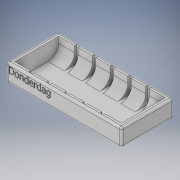
# Autodesk Inventor part: bakje woensdag
Saved by Autodesk Inventor 2019 (Build 230136000, 136)
## iProperties
Created: 2020-10-20
Part Number: bakje woensdag
Material: Generic
Document SubType Name: Modeling
Designer: daanswinters
Density: 1 g/cm^3
Appearance: Default
Author: daanswinters
Autodesk Inventor part; units mm, degrees
ref_plane "YZ Plane" through (0, 0, 0) normal (1, 0, 0) x (0, 1, 0)
ref_plane "XZ Plane" through (0, 0, 0) normal (0, 1, 0) x (-1, 0, 0)
ref_plane "XY Plane" through (0, 0, 0) normal (0, 0, 1) x (1, 0, 0)
sketch "Sketch1" plane through (0, 0, 0) normal (0, 0, 1) x (1, 0, 0)
  line L0 (55, -8.5) -> (-55, -8.5)
  line L1 (-55, -8.5) -> (-55, 8.5)
  line L2 (-55, 8.5) -> (55, 8.5)
  line L3 (55, 8.5) -> (55, -8.5)
  line L4 (55, -8.5) -> (-55, 8.5) construction
  line L5 (-55, -8.5) -> (55, 8.5) construction
  point P0 (0, 0)
  dimension "d0" = 110
  dimension "d1" = 17
  constraints: 12 end point, 2 midpoint, 2 parallel, 1 horizontal, 1 perpendicular
  measures "d0" distance of L1.end L2.end
  measures "d1" distance of L0.end L1.end
extrude "Extrusion1" add sketch "Sketch1" along normal blind 50
sketch "Sketch2" plane through (-55, 8.5, 0) normal (0, 1, 0) x (1, 0, 0)
  line L0 (0, 0) -> (0, -50) projected
  line L1 (110, -50) -> (0, -50)
  line L2 (0, -50) -> (0, 0)
  line L3 (0, 0) -> (110, 0)
  line L4 (110, 0) -> (110, -50)
  line L5 (110, -50) -> (0, 0) construction
  line L6 (0, -50) -> (110, 0) construction
  line L7 (106, -46) -> (106, -4)
  line L8 (4, -4) -> (4, -46)
  line L9 (56.15, -2) -> (53.85, -2)
  line L10 (53.85, -48) -> (56.15, -48)
  line L11 (56.15, -2) -> (53.85, -48) construction
  line L12 (53.85, -2) -> (56.15, -48) construction
  line L13 (73.15, -2) -> (70.85, -2)
  line L14 (70.85, -48) -> (73.15, -48)
  line L15 (73.15, -2) -> (70.85, -48) construction
  line L16 (70.85, -2) -> (73.15, -48) construction
  line L17 (0, -25) -> (110, -25) construction
  line L18 (87.85, -2) -> (90.15, -2)
  line L19 (90.15, -48) -> (87.85, -48)
  line L20 (87.85, -2) -> (90.15, -48) construction
  line L21 (90.15, -2) -> (87.85, -48) construction
  line L22 (36.85, -2) -> (39.15, -2)
  line L23 (39.15, -48) -> (36.85, -48)
  line L24 (36.85, -2) -> (39.15, -48) construction
  line L25 (39.15, -2) -> (36.85, -48) construction
  line L26 (19.85, -2) -> (22.15, -2)
  line L27 (22.15, -48) -> (19.85, -48)
  line L28 (19.85, -2) -> (22.15, -48) construction
  line L29 (22.15, -2) -> (19.85, -48) construction
  line L30 (90.15, -2) -> (90.15, -4)
  line L31 (90.15, -46) -> (90.15, -48)
  line L32 (87.85, -48) -> (87.85, -46)
  line L33 (87.85, -4) -> (87.85, -2)
  line L34 (73.15, -48) -> (73.15, -46)
  line L35 (73.15, -4) -> (73.15, -2)
  line L36 (70.85, -2) -> (70.85, -4)
  line L37 (70.85, -46) -> (70.85, -48)
  line L38 (56.15, -4) -> (56.15, -2)
  line L39 (53.85, -2) -> (53.85, -4)
  line L40 (53.85, -46) -> (53.85, -48)
  line L41 (56.15, -48) -> (56.15, -46)
  line L42 (39.15, -2) -> (39.15, -4)
  line L43 (39.15, -46) -> (39.15, -48)
  line L44 (36.85, -48) -> (36.85, -46)
  line L45 (36.85, -4) -> (36.85, -2)
  line L46 (22.15, -2) -> (22.15, -4)
  line L47 (19.85, -48) -> (19.85, -46)
  line L48 (19.85, -4) -> (19.85, -2)
  line L49 (22.15, -46) -> (22.15, -48)
  line L50 (4, -46) -> (19.95, -46)
  line L51 (22.05, -46) -> (36.95, -46)
  line L52 (39.05, -46) -> (53.95, -46)
  line L53 (56.05, -46) -> (70.95, -46)
  line L54 (73.05, -46) -> (87.95, -46)
  line L55 (90.05, -46) -> (106, -46)
  line L56 (106, -4) -> (90.05, -4)
  line L57 (87.95, -4) -> (73.05, -4)
  line L58 (70.95, -4) -> (56.05, -4)
  line L59 (53.95, -4) -> (39.05, -4)
  line L60 (36.95, -4) -> (22.05, -4)
  line L61 (19.95, -4) -> (4, -4)
  point P0 (55, 0)
  point P1 (55, -25)
  point P2 (72, -25)
  point P3 (89, -25)
  point P4 (38, -25)
  point P5 (21, -25)
  dimension "d4" = 65.556
  dimension "d5" = 110
  dimension "d7" = 2.3
  dimension "d8" = 46
  dimension "d9" = 2.3
  dimension "d10" = 46
  dimension "d11" = 0
  dimension "d12" = 2.3
  dimension "d13" = 46
  dimension "d14" = 2.3
  dimension "d15" = 46
  dimension "d16" = 2.3
  dimension "d17" = 46
  dimension "d18" = 17
  dimension "d19" = 17
  dimension "d20" = 17
  dimension "d21" = 17
  dimension "d22" = 2.862
  dimension "d23" = 2.862
  dimension "d24" = 106
  dimension "d25" = 4
  dimension "d26" = 42
  dimension "d27" = 2
  dimension "d28" = 0
  dimension "d29" = 42
  dimension "d30" = 0
  dimension "d31" = 42
  dimension "d32" = 0
  dimension "d33" = 42
  dimension "d34" = 0
  dimension "d35" = 42
  dimension "d36" = 0
  dimension "d37" = 42
  constraints: 122 end point, 73 parallel, 43 point on line, 17 perpendicular, 14 midpoint, 6 horizontal
  measures "d4" angle of L5 L0
  measures "d5" distance between parallel lines of L4 L0
  measures "d7" distance of L10.end L10.start
  measures "d8" distance of L10.start L9.end
  measures "d9" distance of L14.end L14.start
  measures "d10" distance of L14.start L13.end
  measures "d11" distance from line of L17 point (72, -25)
  measures "d12" distance of L19.start L19.end
  measures "d13" distance of L18.end L19.start
  measures "d14" distance of L23.start L23.end
  measures "d15" distance of L22.end L23.start
  measures "d16" distance of L27.start L27.end
  measures "d17" distance of L26.end L27.start
  measures "d18" distance of point (72, -25) point (55, -25)
  measures "d19" distance of point (89, -25) point (72, -25)
  measures "d20" distance of point (38, -25) point (55, -25)
  measures "d21" distance of point (21, -25) point (38, -25)
  measures "d22" angle of L0 L20
  measures "d23" angle of L0 L21
  measures "d24" distance between parallel lines of L7 L0
  measures "d25" distance between parallel lines of L8 L0
  measures "d26" distance between parallel lines of L56 L55
  measures "d27" distance between parallel lines of L56 L18
  measures "d28" distance between parallel lines of L56 L57
  measures "d29" distance between parallel lines of L56 L54
  measures "d30" distance between parallel lines of L56 L58
  measures "d31" distance between parallel lines of L56 L53
  measures "d32" distance between parallel lines of L56 L59
  measures "d33" distance between parallel lines of L56 L52
  measures "d34" distance between parallel lines of L56 L60
  measures "d35" distance between parallel lines of L56 L51
  measures "d36" distance between parallel lines of L56 L61
  measures "d37" distance between parallel lines of L56 L50
extrude "Extrusion2" cut sketch "Sketch2" against normal blind 16 contours L55 L31 L19 L32 L54 L34 L14 L37 L53 L41 L10 L40 L52 L43 L23 L44 L51 L49 L27 L47 L50 L8 L61 L48 L26 L46 L60 L45 L22 L42 L59 L39 L9 L38 L58 L36 L13 L35 L57 L33 L18 L30 L56 L7
fillet "Fillet1" radius 2 12 edges at (-55, 0, 50) (-55, 0, 0) (55, 0, 50) (55, 0, 0) (0, 8.5, 50) (-55, 8.5, 25) (0, 8.5, 0) (55, 8.5, 25) (55, -8.5, 25) (0, -8.5, 50) (-55, -8.5, 25) (0, -8.5, 0)
fillet "Fillet2" radius 10 6 edges at (-43.075, -7.5, 4) (-25.5, -7.5, 4) (-8.5, -7.5, 4) (8.5, -7.5, 4) (25.5, -7.5, 4) (43.075, -7.5, 4)
sketch "Sketch3" plane through (35.15, 8.5, 4) normal (0, 1, 0) x (1, 0, 0)
  line L0 (-70.3, -44) -> (-70.3, -42) projected
  line L1 (-51, 2) -> (-53.3, 2)
  line L2 (-34, 2) -> (-34, 0) projected
  line L3 (-36.3, -44) -> (-36.3, -42) projected
  line L4 (-19.3, -44) -> (-19.3, -42) projected
  line L5 (-2.3, -44) -> (-2.3, -42) projected
  line L6 (0, 2) -> (0, 0) projected
  line L7 (-19.8, 2) -> (-16.5, 2)
  line L8 (-16.5, 2) -> (-16.5, -44)
  line L9 (-16.5, -44) -> (-19.8, -44)
  line L10 (-19.8, -44) -> (-19.8, 2)
  line L11 (-19.8, 2) -> (-16.5, -44) construction
  line L12 (-16.5, 2) -> (-19.8, -44) construction
  line L13 (-2.8, -44) -> (0.5, -44)
  line L14 (0.5, -44) -> (0.5, 2)
  line L15 (0.5, 2) -> (-2.8, 2)
  line L16 (-2.8, 2) -> (-2.8, -44)
  line L17 (-2.8, -44) -> (0.5, 2) construction
  line L18 (0.5, -44) -> (-2.8, 2) construction
  line L19 (-36.8, -44) -> (-33.5, -44)
  line L20 (-33.5, -44) -> (-33.5, 2)
  line L21 (-33.5, 2) -> (-36.8, 2)
  line L22 (-36.8, 2) -> (-36.8, -44)
  line L23 (-36.8, -44) -> (-33.5, 2) construction
  line L24 (-33.5, -44) -> (-36.8, 2) construction
  line L25 (-51, 2) -> (-36.3, 2) projected
  line L26 (-53.8, -44) -> (-50.5, -44)
  line L27 (-50.5, -44) -> (-50.5, 2)
  line L28 (-50.5, 2) -> (-53.8, 2)
  line L29 (-53.8, 2) -> (-53.8, -44)
  line L30 (-53.8, -44) -> (-50.5, 2) construction
  line L31 (-50.5, -44) -> (-53.8, 2) construction
  line L32 (-53.3, -44) -> (-68, -44) projected
  line L33 (-70.8, 2) -> (-67.5, 2)
  line L34 (-67.5, 2) -> (-67.5, -44)
  line L35 (-67.5, -44) -> (-70.8, -44)
  line L36 (-70.8, -44) -> (-70.8, 2)
  line L37 (-70.8, 2) -> (-67.5, -44) construction
  line L38 (-67.5, 2) -> (-70.8, -44) construction
  point P0 (-35.15, 4)
  point P1 (-68, 2)
  point P2 (-17, 2)
  point P3 (-18.15, -21)
  point P4 (-1.15, -21)
  point P5 (-35.15, -21)
  point P6 (-52.15, -21)
  point P7 (-69.15, -21)
  dimension "d42" = 3.3
  dimension "d43" = 46
  dimension "d44" = 3.3
  dimension "d45" = 3.3
  dimension "d46" = 3.3
  dimension "d47" = 3.3
  dimension "d48" = 90
  dimension "d49" = 0.5
  dimension "d50" = 16.5
  dimension "d51" = 33.5
  dimension "d52" = 50.5
  dimension "d53" = 67.5
  dimension "d54" = 46
  dimension "d55" = 0
  dimension "d56" = 53.3
  constraints: 62 end point, 14 parallel, 10 midpoint, 5 horizontal, 5 perpendicular, 3 point on line
  measures "d42" distance of L8.end L9.end
  measures "d43" distance of L7.end L8.end
  measures "d44" distance of L15.end L14.end
  measures "d45" distance of L21.end L20.end
  measures "d46" distance of L28.end L27.end
  measures "d47" distance of L34.end L35.end
  measures "d48" angle of L6 L1
  measures "d49" distance between parallel lines of L6 L14
  measures "d50" distance between parallel lines of L6 L8
  measures "d51" distance between parallel lines of L6 L20
  measures "d52" distance between parallel lines of L6 L27
  measures "d53" distance between parallel lines of L6 L34
  measures "d54" distance between parallel lines of L25 L9
  measures "d55" distance between parallel lines of L15 L25
  measures "d56" distance from line of L1.end L6
extrude "Extrusion3" cut sketch "Sketch3" against normal blind 16
sketch "Sketch4" plane through (0, 0, 50) normal (0, 0, 1) x (1, 0, 0)
  line L0 (-52.9749, 6.5012) -> (53.0345, 6.5012) construction
  line L1 (53.0345, 6.5012) -> (53.0345, -6.5247) construction
  line L2 (53.0345, -6.5247) -> (-52.9749, -6.5247) construction
  line L3 (-52.9749, -6.5247) -> (-52.9749, 6.5012) construction
  spline S0 degree 2 poles (-47.5472, 3.1744) (-47.5472, 2.339) (-48.2244, 0.9944) (-48.7929, 0.6188) knots 0 0 0 1 2 2 2
  spline S1 degree 2 poles (-48.7929, 0.6188) (-49.2576, 0.3271) (-50.2116, 0.1294) (-50.9531, 0.1294) knots 0 0 0 1 2 2 2
  line L4 (-50.9531, 0.1294) -> (-52.357, 0.1294)
  line L5 (-52.357, 0.1294) -> (-52.357, 6.2294)
  line L6 (-52.357, 6.2294) -> (-50.968, 6.2294)
  spline S2 degree 2 poles (-50.968, 6.2294) (-50.1078, 6.2294) (-49.1291, 5.9723) (-48.783, 5.7449) knots 0 0 0 1 2 2 2
  spline S3 degree 2 poles (-48.783, 5.7449) (-48.1948, 5.3544) (-47.5472, 4.0642) (-47.5472, 3.1744) knots 0 0 0 1 2 2 2
  spline S4 degree 2 poles (-48.3925, 3.1843) (-48.3925, 3.8863) (-48.8572, 4.8799) (-49.3169, 5.1616) knots 0 0 0 1 2 2 2
  spline S5 degree 2 poles (-49.3169, 5.1616) (-49.6432, 5.3544) (-50.3797, 5.5274) (-50.9284, 5.5274) knots 0 0 0 1 2 2 2
  line L7 (-50.9284, 5.5274) -> (-51.5463, 5.5274)
  line L8 (-51.5463, 5.5274) -> (-51.5463, 0.8313)
  line L9 (-51.5463, 0.8313) -> (-50.9284, 0.8313)
  spline S6 degree 2 poles (-50.9284, 0.8313) (-50.3896, 0.8313) (-49.574, 1.0043) (-49.2428, 1.2367) knots 0 0 0 1 2 2 2
  spline S7 degree 2 poles (-49.2428, 1.2367) (-48.8176, 1.5234) (-48.3925, 2.4725) (-48.3925, 3.1843) knots 0 0 0 1 2 2 2
  spline S8 degree 2 poles (-42.9648, 2.4181) (-42.9648, 1.2614) (-44.077, 0.0008) (-45.0064, 0.0008) knots 0 0 0 1 2 2 2
  spline S9 degree 2 poles (-45.0064, 0.0008) (-45.9604, 0.0008) (-47.0529, 1.3009) (-47.0529, 2.4181) knots 0 0 0 1 2 2 2
  spline S10 degree 2 poles (-47.0529, 2.4181) (-47.0529, 3.5649) (-45.9258, 4.8354) (-45.0064, 4.8354) knots 0 0 0 1 2 2 2
  spline S11 degree 2 poles (-45.0064, 4.8354) (-44.077, 4.8354) (-42.9648, 3.5699) (-42.9648, 2.4181) knots 0 0 0 1 2 2 2
  spline S12 degree 2 poles (-43.7607, 2.4181) (-43.7607, 3.3079) (-44.4082, 4.173) (-45.0064, 4.173) knots 0 0 0 1 2 2 2
  spline S13 degree 2 poles (-45.0064, 4.173) (-45.6045, 4.173) (-46.257, 3.3079) (-46.257, 2.4181) knots 0 0 0 1 2 2 2
  spline S14 degree 2 poles (-46.257, 2.4181) (-46.257, 1.553) (-45.6045, 0.6632) (-45.0064, 0.6632) knots 0 0 0 1 2 2 2
  spline S15 degree 2 poles (-45.0064, 0.6632) (-44.4132, 0.6632) (-43.7607, 1.5382) (-43.7607, 2.4181) knots 0 0 0 1 2 2 2
  line L10 (-38.5801, 0.1294) -> (-39.3513, 0.1294)
  line L11 (-39.3513, 0.1294) -> (-39.3513, 2.7394)
  spline S16 degree 2 poles (-39.3513, 2.7394) (-39.3513, 3.0558) (-39.4106, 3.5995) (-39.4996, 3.7627) knots 0 0 0 1 2 2 2
  spline S17 degree 2 poles (-39.4996, 3.7627) (-39.5935, 3.9357) (-39.9296, 4.1038) (-40.2163, 4.1038) knots 0 0 0 1 2 2 2
  spline S18 degree 2 poles (-40.2163, 4.1038) (-40.503, 4.1038) (-41.1111, 3.7973) (-41.4027, 3.5501) knots 0 0 0 1 2 2 2
  line L12 (-41.4027, 3.5501) -> (-41.4027, 0.1294)
  line L13 (-41.4027, 0.1294) -> (-42.1739, 0.1294)
  line L14 (-42.1739, 0.1294) -> (-42.1739, 4.7068)
  line L15 (-42.1739, 4.7068) -> (-41.4027, 4.7068)
  line L16 (-41.4027, 4.7068) -> (-41.4027, 4.1977)
  spline S19 degree 2 poles (-41.4027, 4.1977) (-41.0567, 4.5091) (-40.3894, 4.8354) (-40.0137, 4.8354) knots 0 0 0 1 2 2 2
  spline S20 degree 2 poles (-40.0137, 4.8354) (-39.3414, 4.8354) (-38.5801, 3.9456) (-38.5801, 3.1003) knots 0 0 0 1 2 2 2
  line L17 (-38.5801, 3.1003) -> (-38.5801, 0.1294)
  line L18 (-33.9779, 0.1294) -> (-34.7491, 0.1294)
  line L19 (-34.7491, 0.1294) -> (-34.7491, 0.594)
  spline S21 degree 2 poles (-34.7491, 0.594) (-34.927, 0.4457) (-35.189, 0.248) (-35.367, 0.164) knots 0 0 0 1 2 2 2
  spline S22 degree 2 poles (-35.367, 0.164) (-35.5301, 0.0849) (-35.8811, 0.0008) (-36.1134, 0.0008) knots 0 0 0 1 2 2 2
  spline S23 degree 2 poles (-36.1134, 0.0008) (-36.4891, 0.0008) (-37.1218, 0.3123) (-37.3443, 0.6138) knots 0 0 0 1 2 2 2
  spline S24 degree 2 poles (-37.3443, 0.6138) (-37.5667, 0.9153) (-37.8139, 1.8051) (-37.8139, 2.3835) knots 0 0 0 1 2 2 2
  spline S25 degree 2 poles (-37.8139, 2.3835) (-37.8139, 2.9866) (-37.5025, 3.8665) (-37.2306, 4.1977) knots 0 0 0 1 2 2 2
  spline S26 degree 2 poles (-37.2306, 4.1977) (-36.9785, 4.4943) (-36.2716, 4.8354) (-35.8811, 4.8354) knots 0 0 0 1 2 2 2
  spline S27 degree 2 poles (-35.8811, 4.8354) (-35.54, 4.8354) (-35.0308, 4.6821) (-34.7491, 4.5239) knots 0 0 0 1 2 2 2
  line L20 (-34.7491, 4.5239) -> (-34.7491, 6.5012)
  line L21 (-34.7491, 6.5012) -> (-33.9779, 6.5012)
  line L22 (-33.9779, 6.5012) -> (-33.9779, 0.1294)
  line L23 (-34.7491, 1.2416) -> (-34.7491, 3.8863)
  spline S28 degree 2 poles (-34.7491, 3.8863) (-35.0358, 4.0247) (-35.4906, 4.1285) (-35.7526, 4.1285) knots 0 0 0 1 2 2 2
  spline S29 degree 2 poles (-35.7526, 4.1285) (-36.3458, 4.1285) (-37.018, 3.2387) (-37.018, 2.3983) knots 0 0 0 1 2 2 2
  spline S30 degree 2 poles (-37.018, 2.3983) (-37.018, 1.5876) (-36.5039, 0.7324) (-35.9355, 0.7324) knots 0 0 0 1 2 2 2
  spline S31 degree 2 poles (-35.9355, 0.7324) (-35.6339, 0.7324) (-35.021, 1.0093) (-34.7491, 1.2416) knots 0 0 0 1 2 2 2
  spline S32 degree 2 poles (-30.8735, 0.0256) (-31.971, 0.0256) (-33.1771, 1.2564) (-33.1771, 2.3934) knots 0 0 0 1 2 2 2
  spline S33 degree 2 poles (-33.1771, 2.3934) (-33.1771, 3.5106) (-32.0056, 4.8354) (-31.0614, 4.8354) knots 0 0 0 1 2 2 2
  spline S34 degree 2 poles (-31.0614, 4.8354) (-30.6363, 4.8354) (-29.9788, 4.5882) (-29.7366, 4.3262) knots 0 0 0 1 2 2 2
  spline S35 degree 2 poles (-29.7366, 4.3262) (-29.4894, 4.0642) (-29.2274, 3.3079) (-29.2274, 2.7592) knots 0 0 0 1 2 2 2
  line L24 (-29.2274, 2.7592) -> (-29.2274, 2.339)
  line L25 (-29.2274, 2.339) -> (-32.3961, 2.339)
  spline S36 degree 2 poles (-32.3961, 2.339) (-32.3961, 1.5431) (-31.5953, 0.6978) (-30.8834, 0.6978) knots 0 0 0 1 2 2 2
  spline S37 degree 2 poles (-30.8834, 0.6978) (-30.6313, 0.6978) (-30.1419, 0.8115) (-29.9442, 0.9005) knots 0 0 0 1 2 2 2
  spline S38 degree 2 poles (-29.9442, 0.9005) (-29.7366, 0.9994) (-29.4499, 1.1724) (-29.356, 1.2515) knots 0 0 0 1 2 2 2
  line L26 (-29.356, 1.2515) -> (-29.3115, 1.2515)
  line L27 (-29.3115, 1.2515) -> (-29.3115, 0.4111)
  spline S39 degree 2 poles (-29.3115, 0.4111) (-29.4449, 0.3568) (-29.8503, 0.1986) (-30.0085, 0.1541) knots 0 0 0 1 2 2 2
  spline S40 degree 2 poles (-30.0085, 0.1541) (-30.2309, 0.0898) (-30.5967, 0.0256) (-30.8735, 0.0256) knots 0 0 0 1 2 2 2
  spline S41 degree 2 poles (-29.9788, 2.9273) (-29.9887, 3.2387) (-30.1172, 3.6935) (-30.2408, 3.8467) knots 0 0 0 1 2 2 2
  spline S42 degree 2 poles (-30.2408, 3.8467) (-30.3743, 4.0197) (-30.7945, 4.2026) (-31.1059, 4.2026) knots 0 0 0 1 2 2 2
  spline S43 degree 2 poles (-31.1059, 4.2026) (-31.4124, 4.2026) (-31.8424, 4.0197) (-32.0204, 3.8418) knots 0 0 0 1 2 2 2
  spline S44 degree 2 poles (-32.0204, 3.8418) (-32.1934, 3.6589) (-32.3714, 3.2189) (-32.3961, 2.9273) knots 0 0 0 1 2 2 2
  line L28 (-32.3961, 2.9273) -> (-29.9788, 2.9273)
  line L29 (-26.0193, 3.8813) -> (-26.0588, 3.8813)
  spline S45 degree 2 poles (-26.0588, 3.8813) (-26.1478, 3.906) (-26.3406, 3.9159) (-26.474, 3.9159) knots 0 0 0 1 2 2 2
  spline S46 degree 2 poles (-26.474, 3.9159) (-26.7855, 3.9159) (-27.3984, 3.644) (-27.6753, 3.3771) knots 0 0 0 1 2 2 2
  line L30 (-27.6753, 3.3771) -> (-27.6753, 0.1294)
  line L31 (-27.6753, 0.1294) -> (-28.4464, 0.1294)
  line L32 (-28.4464, 0.1294) -> (-28.4464, 4.7068)
  line L33 (-28.4464, 4.7068) -> (-27.6753, 4.7068)
  line L34 (-27.6753, 4.7068) -> (-27.6753, 4.0247)
  spline S47 degree 2 poles (-27.6753, 4.0247) (-27.2551, 4.4004) (-26.6273, 4.7068) (-26.3307, 4.7068) knots 0 0 0 1 2 2 2
  spline S48 degree 2 poles (-26.3307, 4.7068) (-26.212, 4.7068) (-26.0934, 4.697) (-26.0193, 4.6821) knots 0 0 0 1 2 2 2
  line L35 (-26.0193, 4.6821) -> (-26.0193, 3.8813)
  line L36 (-21.9015, 0.1294) -> (-22.6727, 0.1294)
  line L37 (-22.6727, 0.1294) -> (-22.6727, 0.594)
  spline S49 degree 2 poles (-22.6727, 0.594) (-22.8506, 0.4457) (-23.1126, 0.248) (-23.2906, 0.164) knots 0 0 0 1 2 2 2
  spline S50 degree 2 poles (-23.2906, 0.164) (-23.4537, 0.0849) (-23.8047, 0.0008) (-24.037, 0.0008) knots 0 0 0 1 2 2 2
  spline S51 degree 2 poles (-24.037, 0.0008) (-24.4127, 0.0008) (-25.0454, 0.3123) (-25.2679, 0.6138) knots 0 0 0 1 2 2 2
  spline S52 degree 2 poles (-25.2679, 0.6138) (-25.4903, 0.9153) (-25.7375, 1.8051) (-25.7375, 2.3835) knots 0 0 0 1 2 2 2
  spline S53 degree 2 poles (-25.7375, 2.3835) (-25.7375, 2.9866) (-25.4261, 3.8665) (-25.1542, 4.1977) knots 0 0 0 1 2 2 2
  spline S54 degree 2 poles (-25.1542, 4.1977) (-24.9021, 4.4943) (-24.1952, 4.8354) (-23.8047, 4.8354) knots 0 0 0 1 2 2 2
  spline S55 degree 2 poles (-23.8047, 4.8354) (-23.4636, 4.8354) (-22.9544, 4.6821) (-22.6727, 4.5239) knots 0 0 0 1 2 2 2
  line L38 (-22.6727, 4.5239) -> (-22.6727, 6.5012)
  line L39 (-22.6727, 6.5012) -> (-21.9015, 6.5012)
  line L40 (-21.9015, 6.5012) -> (-21.9015, 0.1294)
  line L41 (-22.6727, 1.2416) -> (-22.6727, 3.8863)
  spline S56 degree 2 poles (-22.6727, 3.8863) (-22.9594, 4.0247) (-23.4141, 4.1285) (-23.6761, 4.1285) knots 0 0 0 1 2 2 2
  spline S57 degree 2 poles (-23.6761, 4.1285) (-24.2693, 4.1285) (-24.9416, 3.2387) (-24.9416, 2.3983) knots 0 0 0 1 2 2 2
  spline S58 degree 2 poles (-24.9416, 2.3983) (-24.9416, 1.5876) (-24.4275, 0.7324) (-23.859, 0.7324) knots 0 0 0 1 2 2 2
  spline S59 degree 2 poles (-23.859, 0.7324) (-23.5575, 0.7324) (-22.9445, 1.0093) (-22.6727, 1.2416) knots 0 0 0 1 2 2 2
  spline S60 degree 2 poles (-18.2336, 0.6138) (-18.3275, 0.5446) (-18.6439, 0.2974) (-18.7922, 0.2233) knots 0 0 0 1 2 2 2
  spline S61 degree 2 poles (-18.7922, 0.2233) (-18.9949, 0.1145) (-19.3755, 0.0008) (-19.7215, 0.0008) knots 0 0 0 1 2 2 2
  spline S62 degree 2 poles (-19.7215, 0.0008) (-20.0033, 0.0008) (-20.5124, 0.2134) (-20.7052, 0.4062) knots 0 0 0 1 2 2 2
  spline S63 degree 2 poles (-20.7052, 0.4062) (-20.8881, 0.594) (-21.1106, 1.1477) (-21.1106, 1.4542) knots 0 0 0 1 2 2 2
  spline S64 degree 2 poles (-21.1106, 1.4542) (-21.1106, 1.9287) (-20.7102, 2.601) (-20.2752, 2.7938) knots 0 0 0 1 2 2 2
  spline S65 degree 2 poles (-20.2752, 2.7938) (-19.8896, 2.9718) (-18.8416, 3.1052) (-18.2336, 3.1398) knots 0 0 0 1 2 2 2
  line L42 (-18.2336, 3.1398) -> (-18.2336, 3.2881)
  spline S66 degree 2 poles (-18.2336, 3.2881) (-18.2336, 3.5551) (-18.3967, 3.8863) (-18.545, 3.9802) knots 0 0 0 1 2 2 2
  spline S67 degree 2 poles (-18.545, 3.9802) (-18.6933, 4.0741) (-19.1184, 4.1334) (-19.3458, 4.1334) knots 0 0 0 1 2 2 2
  spline S68 degree 2 poles (-19.3458, 4.1334) (-19.6128, 4.1334) (-20.3345, 3.9752) (-20.6953, 3.822) knots 0 0 0 1 2 2 2
  line L43 (-20.6953, 3.822) -> (-20.7398, 3.822)
  line L44 (-20.7398, 3.822) -> (-20.7398, 4.608)
  spline S69 degree 2 poles (-20.7398, 4.608) (-20.5273, 4.6673) (-19.7314, 4.8156) (-19.3409, 4.8156) knots 0 0 0 1 2 2 2
  spline S70 degree 2 poles (-19.3409, 4.8156) (-18.8663, 4.8156) (-18.2188, 4.6673) (-17.9617, 4.4745) knots 0 0 0 1 2 2 2
  spline S71 degree 2 poles (-17.9617, 4.4745) (-17.7096, 4.2867) (-17.4624, 3.6885) (-17.4624, 3.2585) knots 0 0 0 1 2 2 2
  line L45 (-17.4624, 3.2585) -> (-17.4624, 0.1294)
  line L46 (-17.4624, 0.1294) -> (-18.2336, 0.1294)
  line L47 (-18.2336, 0.1294) -> (-18.2336, 0.6138)
  line L48 (-18.2336, 1.2564) -> (-18.2336, 2.5269)
  spline S72 degree 2 poles (-18.2336, 2.5269) (-18.5104, 2.5021) (-19.3458, 2.4181) (-19.6078, 2.339) knots 0 0 0 1 2 2 2
  spline S73 degree 2 poles (-19.6078, 2.339) (-19.9143, 2.2451) (-20.3147, 1.8546) (-20.3147, 1.5085) knots 0 0 0 1 2 2 2
  spline S74 degree 2 poles (-20.3147, 1.5085) (-20.3147, 1.1131) (-19.8698, 0.7127) (-19.4447, 0.7127) knots 0 0 0 1 2 2 2
  spline S75 degree 2 poles (-19.4447, 0.7127) (-19.0838, 0.7127) (-18.4906, 1.0241) (-18.2336, 1.2564) knots 0 0 0 1 2 2 2
  spline S76 degree 2 poles (-16.2167, -0.6022) (-16.1376, -0.6368) (-15.8361, -0.7456) (-15.6433, -0.7901) knots 0 0 0 1 2 2 2
  spline S77 degree 2 poles (-15.6433, -0.7901) (-15.4308, -0.8445) (-15.0699, -0.9087) (-14.8573, -0.9087) knots 0 0 0 1 2 2 2
  spline S78 degree 2 poles (-14.8573, -0.9087) (-14.5014, -0.9087) (-14.0071, -0.7209) (-13.8687, -0.5528) knots 0 0 0 1 2 2 2
  spline S79 degree 2 poles (-13.8687, -0.5528) (-13.7352, -0.3847) (-13.6314, 0.0552) (-13.6314, 0.337) knots 0 0 0 1 2 2 2
  line L49 (-13.6314, 0.337) -> (-13.6314, 0.7374)
  spline S80 degree 2 poles (-13.6314, 0.7374) (-13.9428, 0.4655) (-14.541, 0.2085) (-14.9908, 0.2085) knots 0 0 0 1 2 2 2
  spline S81 degree 2 poles (-14.9908, 0.2085) (-15.7718, 0.2085) (-16.6962, 1.3701) (-16.6962, 2.4626) knots 0 0 0 1 2 2 2
  spline S82 degree 2 poles (-16.6962, 2.4626) (-16.6962, 3.0311) (-16.3749, 3.911) (-16.108, 4.2224) knots 0 0 0 1 2 2 2
  spline S83 degree 2 poles (-16.108, 4.2224) (-15.8509, 4.5141) (-15.1441, 4.8354) (-14.7684, 4.8354) knots 0 0 0 1 2 2 2
  spline S84 degree 2 poles (-14.7684, 4.8354) (-14.4124, 4.8354) (-13.8934, 4.6673) (-13.6314, 4.5141) knots 0 0 0 1 2 2 2
  line L50 (-13.6314, 4.5141) -> (-13.5869, 4.7068)
  line L51 (-13.5869, 4.7068) -> (-12.8603, 4.7068)
  line L52 (-12.8603, 4.7068) -> (-12.8603, 0.6534)
  spline S85 degree 2 poles (-12.8603, 0.6534) (-12.8603, -0.5133) (-13.8736, -1.6008) (-14.9167, -1.6008) knots 0 0 0 1 2 2 2
  spline S86 degree 2 poles (-14.9167, -1.6008) (-15.2528, -1.6008) (-15.9547, -1.492) (-16.2563, -1.403) knots 0 0 0 1 2 2 2
  line L53 (-16.2563, -1.403) -> (-16.2563, -0.6022)
  line L54 (-16.2563, -0.6022) -> (-16.2167, -0.6022)
  line L55 (-13.6314, 1.3701) -> (-13.6314, 3.8863)
  spline S87 degree 2 poles (-13.6314, 3.8863) (-13.9181, 4.0247) (-14.4026, 4.1433) (-14.6448, 4.1433) knots 0 0 0 1 2 2 2
  spline S88 degree 2 poles (-14.6448, 4.1433) (-15.2281, 4.1433) (-15.9004, 3.2832) (-15.9004, 2.4774) knots 0 0 0 1 2 2 2
  spline S89 degree 2 poles (-15.9004, 2.4774) (-15.9004, 1.7162) (-15.3912, 0.9203) (-14.8178, 0.9203) knots 0 0 0 1 2 2 2
  spline S90 degree 2 poles (-14.8178, 0.9203) (-14.5163, 0.9203) (-13.8835, 1.1576) (-13.6314, 1.3701) knots 0 0 0 1 2 2 2
  point P0 (0, 0)
  constraints: 2 other
extrude "Extrusion4" cut sketch "Sketch4" against normal blind 0.5
fillet "Fillet3" radius 10 6 edges at (-43.325, -7.5, 46) (-25.5, -7.5, 46) (-8.5, -7.5, 46) (8.5, -7.5, 46) (25.5, -7.5, 46) (43.325, -7.5, 46)
body "Solid1"
